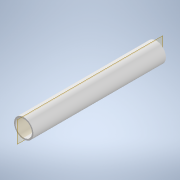
# Autodesk Inventor part: 3inchPvcPipe
Saved by Autodesk Inventor 2022.2 (Build 262287000, 287)
## iProperties
Created: 2021-11-22
Part Number: 3inchPvcPipe
Material: Generic
Document SubType Name: Modeling
Designer: robst
Density: 1 g/cm^3
Appearance: Default
Author: robst
Autodesk Inventor part; units mm, degrees
ref_plane "XZ Plane" through (0, 0, 0) normal (0, 1, 0) x (-1, 0, 0)
ref_plane "XY Plane" through (0, 0, 0) normal (0, 0, 1) x (1, 0, 0)
sketch "Sketch1" plane through (0, 0, 0) normal (0, 0, 1) x (1, 0, 0)
  circle A0 centre (0, 0) radius 44.45
  circle A1 centre (0, 0) radius 37.9476
  dimension "d0" = 88.9
  dimension "d1" = 75.8952
  constraints: 2 centre point, 2 coincident
  measures "d0" diameter of A0
  measures "d1" diameter of A1
extrude "Extrusion1" add sketch "Sketch1" against normal blind 609.6
equation "\"d0\" = outsideDiameter"
equation "\"d1\" = insideDiameter"
equation "\"insideDiameter\" = 75.8952"
equation "\"outsideDiameter\" = 88.9"
body "Solid1"
